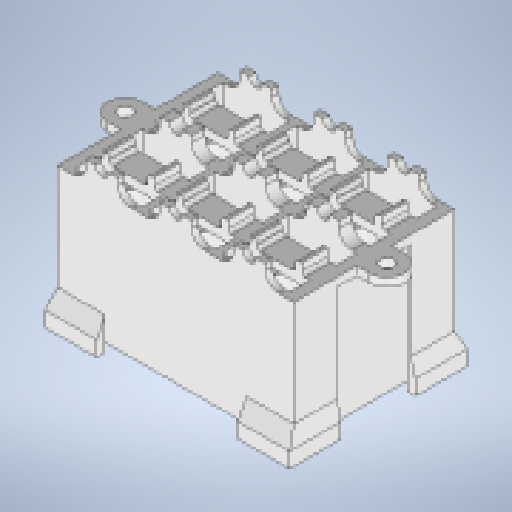
# Autodesk Inventor part: inner_bttm
Saved by Autodesk Inventor 2025.1 (Build 291241000, 241)
## iProperties
Created: 2025-02-27
Part Number: inner_bttm
Material: Generic
Document SubType Name: Modeling
Designer: santiago
Density: 1 g/cm^3
Appearance: Default
Author: santiago
Autodesk Inventor part; units mm, degrees
ref_plane "YZ Plane" through (0, 0, 0) normal (1, 0, 0) x (0, 1, 0)
ref_plane "XZ Plane" through (0, 0, 0) normal (0, 1, 0) x (-1, 0, 0)
ref_plane "XY Plane" through (0, 0, 0) normal (0, 0, 1) x (1, 0, 0)
sketch "Sketch1" plane through (0, 0, 0) normal (0, 1, 0) x (-1, 0, 0)
  line L0 (-7.8, -7.8) -> (7.8, -7.8)
  line L1 (7.8, -7.8) -> (7.8, 7.8)
  line L2 (7.8, 7.8) -> (-7.8, 7.8)
  line L3 (-7.8, 7.8) -> (-7.8, -7.8)
  line L4 (-7.8, -7.8) -> (7.8, 7.8) construction
  line L5 (7.8, -7.8) -> (-7.8, 7.8) construction
  line L6 (9.3, 9.3) -> (-9.3, 9.3)
  line L7 (-9.3, 9.3) -> (-9.3, -9.3)
  line L8 (-9.3, -9.3) -> (9.3, -9.3)
  line L9 (9.3, -9.3) -> (9.3, 9.3)
  line L10 (9.3, 9.3) -> (-9.3, -9.3) construction
  line L11 (-9.3, 9.3) -> (9.3, -9.3) construction
  point P0 (0, 0)
  dimension "d0" = 15.6
  dimension "d1" = 15.6
  dimension "d2" = 18.6
  dimension "d3" = 18.6
  constraints: 24 end point, 4 midpoint, 4 parallel, 2 horizontal, 2 perpendicular
  measures "d0" distance of L2.end L1.end
  measures "d1" distance of L1.end L0.end
  measures "d2" distance of L8.end L7.end
  measures "d3" distance of L7.end L6.end
extrude "Extrusion1" add sketch "Sketch1" along normal blind 30
sketch "Sketch2" plane through (-9.3, 0, 9.3) normal (0, 0, 1) x (1, 0, 0)
  line L0 (18.6, 30) -> (0, 30) projected
  line L1 (5.6, 30) -> (13, 30)
  line L2 (13, 30) -> (13, 34.5)
  line L3 (13, 34.5) -> (5.6, 34.5)
  line L4 (5.6, 34.5) -> (5.6, 30)
  circle A0 centre (9.3, 34.5) radius 1.6
  point P0 (9.3, 0)
  point P1 (9.3, 30)
  point P2 (10.9, 34.5)
  point P3 (7.7, 34.5)
  point P4 (13, 30)
  dimension "d6" = 7.4
  dimension "d7" = 4.5
  dimension "d8" = 3.2
  constraints: 8 end point, 2 midpoint, 2 parallel, 1 centre point, 1 coincident, 1 horizontal, 1 perpendicular, 1 point on line, 1 vertical alignment
  measures "d6" distance of L3.end L2.end
  measures "d7" distance of L2.end L1.end
  measures "d8" diameter of A0
extrude "Extrusion2" add sketch "Sketch2" against normal blind 1.5 contours L0 L4 L3 A0 L2
pattern_linear "Rectangular Pattern1" count 2 spacing 17.1 along (0, 0, -1) of "Extrusion2"
sketch "Sketch3" plane through (0, 30, 0) normal (0, 1, 0) x (1, 0, 0)
  line L0 (-9.3, 9.3) -> (-9.3, -9.3) projected
  line L1 (9.3, 3) -> (-9.3, 3)
  line L2 (-9.3, 3) -> (-9.3, -3)
  line L3 (-9.3, -3) -> (9.3, -3)
  line L4 (9.3, -3) -> (9.3, 3)
  line L5 (9.3, 3) -> (-9.3, -3) construction
  line L6 (-9.3, 3) -> (9.3, -3) construction
  point P0 (0, 0)
  dimension "d14" = 6
  constraints: 12 end point, 2 midpoint, 2 parallel, 1 horizontal, 1 perpendicular, 1 point on line
  measures "d14" distance of L2.end L1.end
extrude "Extrusion3" add sketch "Sketch3" against normal blind 2
sketch "Sketch4" plane through (0, 28, 0) normal (0, -1, 0) x (1, 0, 0)
  circle A0 centre (0, 0) radius 2.25
  dimension "d17" = 4.5
  constraints: 1 centre point, 1 coincident
  measures "d17" diameter of A0
extrude "Extrusion4" cut sketch "Sketch4" against normal blind 1.5
fillet "Fillet1" radius 3 4 edges at (-3.7, 30, -8.55) (3.7, 30, -8.55) (3.7, 30, 8.55) (-3.7, 30, 8.55)
sketch "Sketch5" plane through (0, 30, 0) normal (0, 1, 0) x (1, 0, 0)
  line L0 (7.8, 3) -> (-7.8, 3) projected
  line L1 (-7.8, -3) -> (7.8, -3) projected
  line L2 (4.3, 3) -> (5.8, 3)
  line L3 (5.8, 3) -> (5.8, -3)
  line L4 (5.8, -3) -> (4.3, -3)
  line L5 (4.3, -3) -> (4.3, 3)
  line L6 (7.8, 7.8) -> (7.8, 3) projected
  point P0 (0, 0)
  dimension "d33" = 2
  dimension "d34" = 1.5
  constraints: 8 end point, 2 parallel, 2 point on line, 1 horizontal, 1 perpendicular
  measures "d33" distance between parallel lines of L6 L3
  measures "d34" distance between parallel lines of L3 L5
extrude "Extrusion5" add sketch "Sketch5" along normal blind 2.5
sketch "Sketch6" plane through (0, 30, 0) normal (0, 1, 0) x (1, 0, 0)
  line L0 (7.8, -3) -> (-7.8, -3) projected
  line L1 (-7.8, 3) -> (7.8, 3) projected
  line L2 (-6.05, -3) -> (-4.55, -3)
  line L3 (-4.55, -3) -> (-4.55, 3)
  line L4 (-4.55, 3) -> (-6.05, 3)
  line L5 (-6.05, 3) -> (-6.05, -3)
  line L6 (-7.8, 3) -> (-7.8, 7.8) projected
  point P0 (0, 0)
  point P1 (-7.8, 5.4)
  dimension "d37" = 1.5
  dimension "d38" = 1.75
  constraints: 8 end point, 2 parallel, 2 point on line, 1 horizontal, 1 midpoint, 1 perpendicular
  measures "d37" distance of L4.end L3.end
  measures "d38" distance from line of point (-7.8, 5.4) L5
extrude "Extrusion6" add sketch "Sketch6" along normal blind 2
fillet "Fillet2" radius 0.8 6 edges at (5.8, 30, 0) (4.3, 30, 0) (-4.55, 30, 0) (-6.05, 30, 0) (4.3, 32.5, 0) (-4.55, 32, 0)
fillet "Fillet3" radius 0.2 1 edges at (-2.25, 28, 0)
pattern_linear "Rectangular Pattern4" count 3 spacing 17.1 along (-1, 0, 0) count 2 spacing 18.6 along (0, 0, 1) of "Extrusion1", "Extrusion2", "Rectangular Pattern1", "Extrusion3", "Extrusion4", "Fillet1", "Extrusion5", "Extrusion6", "Fillet2", "Fillet3"
ref_plane "Work Plane1" through (7.8, 0, 0) normal (0, 0, -1) x (-1, 0, 0)
ref_plane "Work Plane2" through (-9.3, 0, 18.6) normal (0, 0, -1) x (-1, 0, 0)
chamfer "Chamfer1" distance 3 angle 45 12 edges at (-24.9, 28, 18.6) (-9.3, 28, 18.6) (-26.4, 28, 18.6) (-42, 28, 18.6) (-42, 28, 0) (-26.4, 28, 0) (-9.3, 28, 0) (-24.9, 28, 0) (7.8, 28, 18.6) (-7.8, 28, 18.6) (-7.8, 28, 0) (7.8, 28, 0)
ref_plane "Work Plane3" through (0, 15, 0) normal (0, -1, 0) x (1, 0, 0)
sketch "Sketch8" plane through (0, 15, 0) normal (0, -1, 0) x (1, 0, 0)
  circle A0 centre (0, 18.6) radius 2.45 projected
  circle A1 centre (0, 18.6) radius 5
  line L0 (7.8, 21.6) -> (7.8, 26.4) projected
  line L1 (-7.8, 10.8) -> (7.8, 10.8)
  line L2 (7.8, 10.8) -> (7.8, 26.4)
  line L3 (7.8, 26.4) -> (-7.8, 26.4)
  line L4 (-7.8, 26.4) -> (-7.8, 10.8)
  line L5 (-7.8, 10.8) -> (7.8, 26.4) construction
  line L6 (7.8, 10.8) -> (-7.8, 26.4) construction
  point P0 (0, 0)
  dimension "d59" = 10
  constraints: 12 end point, 2 midpoint, 2 parallel, 1 centre point, 1 coincident, 1 horizontal, 1 perpendicular
  measures "d59" diameter of A1
extrude "Extrusion8" add sketch "Sketch8" along normal mid plane 15 contours L2 L1 L4 L3 L0
pattern_linear "Rectangular Pattern5" count 3 spacing 17.1 along (-1, 0, 0) count 2 spacing 18.6 along (0, 0, -1) of "Extrusion8"
ref_plane "Work Plane5" through (0, 0, 0) normal (0, -1, 0) x (1, 0, 0)
ref_plane "Work Plane4" through (0, 3.75, 0) normal (0, -1, 0) x (1, 0, 0)
sketch "Sketch10" plane through (0, 0, 0) normal (0, -1, 0) x (1, 0, 0)
  line L0 (-43.5, -9.3) -> (-43.5, 27.9) projected
  line L1 (9.3, -9.3) -> (-43.5, -9.3) projected
  line L2 (9.3, 27.9) -> (9.3, -9.3) projected
  line L3 (-43.5, 27.9) -> (9.3, 27.9) projected
  line L4 (-45.5, -11.3) -> (11.3, -11.3)
  line L5 (11.3, -11.3) -> (11.3, 29.9)
  line L6 (11.3, 29.9) -> (-45.5, 29.9)
  line L7 (-45.5, 29.9) -> (-45.5, -11.3)
  line L8 (-45.5, -11.3) -> (11.3, 29.9) construction
  line L9 (11.3, -11.3) -> (-45.5, 29.9) construction
  point P0 (0, 0)
  point P1 (-17.1, 9.3)
  dimension "d70" = 56.8
  dimension "d71" = 41.2
  constraints: 12 end point, 2 midpoint, 2 parallel, 1 horizontal, 1 perpendicular
  measures "d70" distance of L6.end L5.end
  measures "d71" distance of L5.end L4.end
extrude "Extrusion9" add sketch "Sketch10" along normal blind 2 and the other way blind 1.5
sketch "Sketch11" plane through (0, 30, 0) normal (0, 1, 0) x (1, 0, 0)
  circle A0 centre (-47.5, -9.3) radius 1.55 projected
  line L0 (-40.95, -10.6) -> (-40.95, -8) projected
  line L1 (-42.2, -10.6) -> (-40.95, -10.6) projected
  line L2 (-42.2, -26.6) -> (-42.2, -10.6) projected
  line L3 (-40.95, -26.6) -> (-42.2, -26.6) projected
  line L4 (-40.95, -27.9) -> (-40.95, -26.6) projected
  line L5 (-43.5, -27.9) -> (-40.95, -27.9) projected
  line L6 (-43.5, -13.3) -> (-43.5, -27.9) projected
  line L7 (-43.5, -13.3) -> (-47.5, -13.3) projected
  arc A1 (-47.5, -5.3) -> (-47.5, -13.3) centre (-47.5, -9.3) ccw projected
  line L8 (-47.5, -5.3) -> (-43.5, -5.3) projected
  line L9 (-43.5, 9.3) -> (-43.5, -5.3) projected
  line L10 (-40.95, 9.3) -> (-43.5, 9.3) projected
  line L11 (-40.95, 8) -> (-40.95, 9.3) projected
  line L12 (-42.2, 8) -> (-40.95, 8) projected
  line L13 (-42.2, -8) -> (-42.2, 8) projected
  line L14 (-40.95, -8) -> (-42.2, -8) projected
  circle A2 centre (13.3, -9.3) radius 1.55 projected
  line L15 (6.75, 9.3) -> (6.75, 8) projected
  line L16 (9.3, 9.3) -> (6.75, 9.3) projected
  line L17 (9.3, -5.3) -> (9.3, 9.3) projected
  line L18 (9.3, -5.3) -> (13.3, -5.3) projected
  arc A3 (13.3, -13.3) -> (13.3, -5.3) centre (13.3, -9.3) ccw projected
  line L19 (13.3, -13.3) -> (9.3, -13.3) projected
  line L20 (9.3, -27.9) -> (9.3, -13.3) projected
  line L21 (6.75, -27.9) -> (9.3, -27.9) projected
  line L22 (6.75, -26.6) -> (6.75, -27.9) projected
  line L23 (8, -26.6) -> (6.75, -26.6) projected
  line L24 (8, -10.6) -> (8, -26.6) projected
  line L25 (6.75, -10.6) -> (8, -10.6) projected
  line L26 (6.75, -8) -> (6.75, -10.6) projected
  line L27 (8, -8) -> (6.75, -8) projected
  line L28 (8, 8) -> (8, -8) projected
  line L29 (6.75, 8) -> (8, 8) projected
  point P0 (0, 0)
extrude "Extrusion10" add sketch "Sketch11" against normal blind 2
thicken "Thicken1" operation add thickness 1 both sides no extend neighbours no toward (1, 0, 0) faces at (9.3, 10.3333, 1.7667) (9.3, 10.3333, 16.8333)
thicken "Thicken2" operation add thickness 1 both sides no extend neighbours no toward (-1, 0, 0) faces at (-43.5, 10.3333, 7.9667)
chamfer "Chamfer2" distance 2 distance2 4 5 edges at (-44, 1.5, -9.3) (-16.6, 1.5, -9.3) (9.8, 1.5, 27.9) (-17.1, 1.5, 27.9) (-44, 1.5, 27.9) measured on face at (-44, 1.5, -9.8) measured on face at (-17.1, 1.5, 28.4) measured on face at (-16.6, 1.5, -9.8) measured on face at (9.8, 1.5, 28.4) measured on face at (-44, 1.5, 28.4)
chamfer "Chamfer3" distance 1 distance2 4 4 edges at (10.3, 1.5, -10.3) (10.3, 1.5, 0) (10.3, 1.5, 18.6) (10.3, 1.5, 28.8999) measured on face at (10.8, 1.5, 0) measured on face at (10.8, 1.5, -10.3) measured on face at (10.8, 1.5, 18.6) measured on face at (10.8, 1.5, 28.8999)
chamfer "Chamfer4" distance 1 distance2 4 3 edges at (-44.5, 1.5, 28.9) (-44.5, 1.5, 9.3) (-44.5, 1.5, -10.3) measured on face at (-45, 1.5, 9.3) measured on face at (-45, 1.5, 28.9) measured on face at (-45, 1.5, -10.3)
sketch "Sketch13" plane through (0, -2, 0) normal (0, -1, 0) x (1, 0, 0)
  line L0 (-44.5, -9.3) -> (10.3, -9.3) projected
  line L1 (-0.715, -9.3) -> (-0.715, -11.3)
  line L2 (11.3, -11.3) -> (-45.5, -11.3) projected
  line L3 (-33.485, -9.3) -> (-33.485, -11.3)
  line L4 (11.3, -11.3) -> (11.3, 29.9) projected
  line L5 (-45.5, 29.9) -> (-45.5, -11.3) projected
  point P0 (0, 0)
  dimension "d93" = 12.015
  dimension "d94" = 12.015
  constraints: 4 end point, 4 point on line, 1 parallel, 1 vertical
  measures "d93" distance between parallel lines of L4 L1
  measures "d94" distance between parallel lines of L5 L3
extrude "Extrusion11" cut sketch "Sketch13" against normal through all
ref_plane "Work Plane6" through (0, 34.5, 9.3) normal (0, 0, -1) x (-1, 0, 0)
mirror "Mirror1" about plane through (0, 34.5, 9.3) normal (0, 0, -1) of "Extrusion11"
sketch "Sketch14" plane through (-44.5, 28, 13.3) normal (-1, 0, 0) x (0, 0, 1)
  line L0 (8.3, 0) -> (2.3, 0) projected
  line L1 (16.6, -30) -> (-24.6, -30) projected
  line L2 (4.6, 0) -> (-12.6, 0)
  line L3 (-12.6, 0) -> (-12.6, -30)
  line L4 (-12.6, -30) -> (4.6, -30)
  line L5 (4.6, -30) -> (4.6, 0)
  line L6 (0, 2) -> (0, 0) projected
  line L7 (-8, 2) -> (-8, 0) projected
  point P0 (-13.3, -28)
  point P1 (0, 1)
  point P2 (-8, 1)
  point P3 (4.6, -30)
  dimension "d97" = 4.6
  dimension "d98" = 4.6
  constraints: 8 end point, 2 midpoint, 2 parallel, 2 point on line, 1 horizontal, 1 perpendicular
  measures "d97" distance from line of point (0, 1) L5
  measures "d98" distance from line of L3 point (-8, 1)
extrude "Extrusion12" cut sketch "Sketch14" along normal blind 2 and the other way blind 1
ref_plane "Work Plane7" through (-17.1, 28, 5.3) normal (-1, 0, 0) x (0, 0, 1)
mirror "Mirror2" about plane through (-17.1, 28, 5.3) normal (-1, 0, 0) of "Extrusion12"
body "Solid1"
